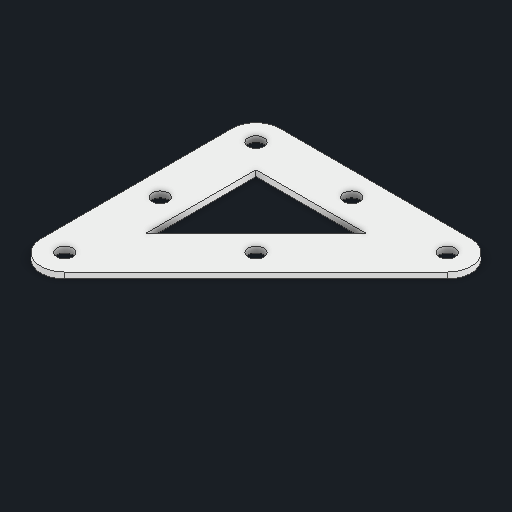
# Autodesk Inventor part: Arm Triangle Gusset
Saved by Autodesk Inventor 2025.1 (Build 291241000, 241)
## iProperties
Created: 2024-10-21
Part Number: Arm Triangle Gusset
Material: Acetal Resin, White
Document SubType Name: Sheet Metal
Designer: averey
Density: 1.425 g/cm^3
Appearance: Smooth - White
Flat Pattern Width: 6.35 cm
Flat Pattern Length: 6.35 cm
Flat Pattern Area: 40.3225 cm^2
Sheet Metal Rule: Default_mm
Sheet Metal Width: 2.500 in
Sheet Metal Length: 2.500 in
Sheet Metal Area: 6.250 in^2
Mass: 4.18559 g
Surface Area: 41.3629 cm^2
Volume: 2.93725 cm^3
Author: averey
Autodesk Inventor part; units mm, degrees
ref_plane "YZ Plane" through (0, 0, 0) normal (1, 0, 0) x (0, 1, 0)
ref_plane "XZ Plane" through (0, 0, 0) normal (0, 1, 0) x (-1, 0, 0)
ref_plane "XY Plane" through (0, 0, 0) normal (0, 0, 1) x (1, 0, 0)
sketch "main" plane through (0, 0, 0) normal (0, 0, 1) x (1, 0, 0)
  circle A0 centre (27.8145, 23.5161) radius 2.0955
  circle A1 centre (27.8145, -27.2839) radius 2.0955
  circle A2 centre (-22.9855, -27.2839) radius 2.0955
  arc A3 (-27.4757, -22.7938) -> (-22.9855, -33.6339) centre (-22.9855, -27.2839) ccw
  arc A4 (27.8145, -33.6339) -> (34.1645, -27.2839) centre (27.8145, -27.2839) ccw
  arc A5 (34.1645, 23.5161) -> (23.3243, 28.0062) centre (27.8145, 23.5161) ccw
  line L0 (34.1645, 23.5161) -> (34.1645, -27.2839)
  line L1 (27.8145, -33.6339) -> (-22.9855, -33.6339)
  line L2 (23.3243, 28.0062) -> (-27.4757, -22.7938)
  line L3 (-7.6553, -20.9339) -> (21.4645, -20.9339)
  line L4 (21.4645, -20.9339) -> (21.4645, 8.1858)
  line L5 (21.4645, 8.1858) -> (-7.6553, -20.9339)
  circle A6 centre (2.4145, -1.8839) radius 2.0955
  point P0 (11.2944, -10.7639)
  dimension "d3" = 4.191
  dimension "d4" = 4.191
  dimension "d5" = 4.191
  dimension "d7" = 12.7
  dimension "d8" = 4.191
  measures "d3" diameter of A1
  measures "d4" diameter of A0
  measures "d5" diameter of A2
  measures "d7" distance between parallel lines of L2 L5
  measures "d8" diameter of A6
sketch "Sketch1" plane through (0, 0, 0) normal (0, 1, 0) x (-1, 0, 0)
  circle A0 centre (-25.4, 0) radius 2.0955
  circle A1 centre (0, 25.4) radius 2.0955
  circle A2 centre (0, 50.8) radius 2.0955
  circle A3 centre (0, 0) radius 2.0955
  circle A4 centre (-50.8, 0) radius 2.0955
  arc A5 (-55.2901, 4.4901) -> (-50.8, -6.35) centre (-50.8, 0) ccw
  arc A6 (0, -6.35) -> (6.35, 0) centre (0, 0) ccw
  arc A7 (6.35, 50.8) -> (-4.4901, 55.2901) centre (0, 50.8) ccw
  line L0 (6.35, 50.8) -> (6.35, 0)
  line L1 (0, -6.35) -> (-50.8, -6.35)
  line L2 (-4.4901, 55.2901) -> (-55.2901, 4.4901)
  line L3 (-35.4697, 6.35) -> (-6.35, 6.35)
  line L4 (-6.35, 6.35) -> (-6.35, 35.4697)
  line L5 (-6.35, 35.4697) -> (-35.4697, 6.35)
  circle A8 centre (-25.4, 25.4) radius 2.0955
  dimension "d2" = 4.191
  dimension "d6" = 4.191
  constraints: 2 centre point, 1 other
  measures "d2" diameter of A0
  measures "d6" diameter of A1
extrude "Extrusion1" add sketch "Sketch1" along normal blind 1.5875
equation "\"BendRadius\" = Thickness"
equation "\"BendReliefWidth\" = Thickness"
equation "\"BendReliefDepth\" = 0.5 * Thickness"
equation "\"CornerReliefSize\" = 4 * Thickness"
equation "\"MinimumRemnant\" = 2 * Thickness"
equation "\"TransitionRadius\" = BendRadius"
equation "\"JacobiRadiusSize\" = BendRadius"
equation "\"GapSize\" = Thickness"
equation "\"Thickness\" = 1.5875"
body "Solid1"
